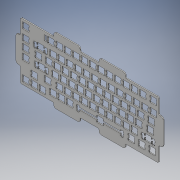
# Autodesk Inventor part: plate
Saved by Autodesk Inventor 2017 (Build 210142000, 142)
## iProperties
Created: 2021-06-16
Part Number: plate
Material: Generic
Document SubType Name: Modeling
Designer: Jack
Density: 1 g/cm^3
Appearance: Default
Author: Jack
Autodesk Inventor part; units mm, degrees
(part 1 of 3)
ref_plane "YZ Plane" through (0, 0, 0) normal (1, 0, 0) x (0, 1, 0)
ref_plane "XZ Plane" through (0, 0, 0) normal (0, 1, 0) x (-1, 0, 0)
ref_plane "XY Plane" through (0, 0, 0) normal (0, 0, 1) x (1, 0, 0)
sketch "Sketch1" plane through (0, 0, 0) normal (0, 1, 0) x (-1, 0, 0)
  line L0 (-149.0682, 63.7581) -> (-78.3822, 63.7581)
  line L1 (163.5067, 60.7579) -> (163.5067, 31.3429)
  line L2 (-152.0562, -63.0674) -> (-152.0562, -33.6571)
  line L3 (143.9807, -46.542) -> (143.9807, -47.5424)
  line L4 (143.9807, -47.5424) -> (143.1797, -47.5424)
  line L5 (143.1797, -47.5424) -> (143.1797, -50.6403)
  line L6 (143.1797, -50.6403) -> (143.9807, -50.6403)
  line L7 (143.9807, -50.6403) -> (143.9807, -56.4418)
  line L8 (143.9807, -56.4418) -> (143.1797, -56.4418)
  line L9 (143.1797, -56.4418) -> (143.1797, -59.5424)
  line L10 (143.1797, -59.5424) -> (143.9807, -59.5424)
  line L11 (143.9807, -59.5424) -> (143.9807, -60.5415)
  line L12 (143.9807, -60.5415) -> (157.9807, -60.5415)
  line L13 (157.9807, -60.5415) -> (157.9807, -59.5424)
  line L14 (157.9807, -59.5424) -> (158.7797, -59.5424)
  line L15 (158.7797, -59.5424) -> (158.7797, -56.4418)
  line L16 (158.7797, -56.4418) -> (157.9807, -56.4418)
  line L17 (157.9807, -56.4418) -> (157.9807, -50.6403)
  line L18 (157.9807, -50.6403) -> (158.7797, -50.6403)
  line L19 (158.7797, -50.6403) -> (158.7797, -47.5424)
  line L20 (158.7797, -47.5424) -> (157.9807, -47.5424)
  line L21 (157.9807, -47.5424) -> (157.9807, -46.542)
  line L22 (157.9807, -46.542) -> (143.9807, -46.542)
  line L23 (124.9307, -46.542) -> (124.9307, -47.5424)
  line L24 (124.9307, -47.5424) -> (124.1297, -47.5424)
  line L25 (124.1297, -47.5424) -> (124.1297, -50.6403)
  line L26 (124.1297, -50.6403) -> (124.9307, -50.6403)
  line L27 (124.9307, -50.6403) -> (124.9307, -56.4418)
  line L28 (124.9307, -56.4418) -> (124.1297, -56.4418)
  line L29 (124.1297, -56.4418) -> (124.1297, -59.5424)
  line L30 (124.1297, -59.5424) -> (124.9307, -59.5424)
  line L31 (124.9307, -59.5424) -> (124.9307, -60.5415)
  line L32 (124.9307, -60.5415) -> (138.9307, -60.5415)
  line L33 (138.9307, -60.5415) -> (138.9307, -59.5424)
  line L34 (138.9307, -59.5424) -> (139.7297, -59.5424)
  line L35 (139.7297, -59.5424) -> (139.7297, -56.4418)
  line L36 (139.7297, -56.4418) -> (138.9307, -56.4418)
  line L37 (138.9307, -56.4418) -> (138.9307, -50.6403)
  line L38 (138.9307, -50.6403) -> (139.7297, -50.6403)
  line L39 (139.7297, -50.6403) -> (139.7297, -47.5424)
  line L40 (139.7297, -47.5424) -> (138.9307, -47.5424)
  line L41 (138.9307, -47.5424) -> (138.9307, -46.542)
  line L42 (138.9307, -46.542) -> (124.9307, -46.542)
  line L43 (105.8807, -46.542) -> (105.8807, -47.5424)
  line L44 (105.8807, -47.5424) -> (105.0797, -47.5424)
  line L45 (105.0797, -47.5424) -> (105.0797, -50.6403)
  line L46 (105.0797, -50.6403) -> (105.8807, -50.6403)
  line L47 (105.8807, -50.6403) -> (105.8807, -56.4418)
  line L48 (105.8807, -56.4418) -> (105.0797, -56.4418)
  line L49 (105.0797, -56.4418) -> (105.0797, -59.5424)
  line L50 (105.0797, -59.5424) -> (105.8807, -59.5424)
  line L51 (105.8807, -59.5424) -> (105.8807, -60.5415)
  line L52 (105.8807, -60.5415) -> (119.8807, -60.5415)
  line L53 (119.8807, -60.5415) -> (119.8807, -59.5424)
  line L54 (119.8807, -59.5424) -> (120.6797, -59.5424)
  line L55 (120.6797, -59.5424) -> (120.6797, -56.4418)
  line L56 (120.6797, -56.4418) -> (119.8807, -56.4418)
  line L57 (119.8807, -56.4418) -> (119.8807, -50.6403)
  line L58 (119.8807, -50.6403) -> (120.6797, -50.6403)
  line L59 (120.6797, -50.6403) -> (120.6797, -47.5424)
  line L60 (120.6797, -47.5424) -> (119.8807, -47.5424)
  line L61 (119.8807, -47.5424) -> (119.8807, -46.542)
  line L62 (119.8807, -46.542) -> (105.8807, -46.542)
  line L63 (-25.0893, -41.7795) -> (-25.0893, -42.7785)
  line L64 (-25.0893, -42.7785) -> (-25.8883, -42.7785)
  line L65 (-25.8883, -42.7785) -> (-25.8883, -45.8791)
  line L66 (-25.8883, -45.8791) -> (-25.0893, -45.8791)
  line L67 (-25.0893, -45.8791) -> (-25.0893, -46.4786)
  line L68 (-25.0893, -46.4786) -> (-64.7132, -46.4786)
  line L69 (-64.7132, -46.4786) -> (-64.7132, -43.2484)
  line L70 (-64.7132, -43.2484) -> (-71.4643, -43.2484)
  line L71 (-71.4643, -43.2484) -> (-71.4643, -46.4786)
  line L72 (-71.4643, -46.4786) -> (-72.2884, -46.4786)
  line L73 (-72.2884, -46.4786) -> (-72.2884, -49.2788)
  line L74 (-72.2884, -49.2788) -> (-71.4643, -49.2788)
  line L75 (-71.4643, -49.2788) -> (-71.4643, -55.5488)
  line L76 (-71.4643, -55.5488) -> (-69.7393, -55.5488)
  line L77 (-69.7393, -55.5488) -> (-69.7393, -56.7491)
  line L78 (-69.7393, -56.7491) -> (-66.4387, -56.7491)
  line L79 (-66.4387, -56.7491) -> (-66.4387, -55.5488)
  line L80 (-66.4387, -55.5488) -> (-64.7132, -55.5488)
  line L81 (-64.7132, -55.5488) -> (-64.7132, -51.0785)
  line L82 (-64.7132, -51.0785) -> (-25.0893, -51.0785)
  line L83 (-25.0893, -51.0785) -> (-25.0893, -51.6793)
  line L84 (-25.0893, -51.6793) -> (-25.8883, -51.6793)
  line L85 (-25.8883, -51.6793) -> (-25.8883, -54.7785)
  line L86 (-25.8883, -54.7785) -> (-25.0893, -54.7785)
  line L87 (-25.0893, -54.7785) -> (-25.0893, -55.779)
  line L88 (-25.0893, -55.779) -> (-11.0883, -55.779)
  line L89 (-11.0883, -55.779) -> (-11.0883, -54.7785)
  line L90 (-11.0883, -54.7785) -> (-10.2893, -54.7785)
  line L91 (-10.2893, -54.7785) -> (-10.2893, -51.6793)
  line L92 (-10.2893, -51.6793) -> (-11.0883, -51.6793)
  line L93 (-11.0883, -51.6793) -> (-11.0883, -51.0785)
  line L94 (-11.0883, -51.0785) -> (28.5357, -51.0785)
  line L95 (28.5357, -51.0785) -> (28.5357, -55.5488)
  line L96 (28.5357, -55.5488) -> (30.2607, -55.5488)
  line L97 (30.2607, -55.5488) -> (30.2607, -56.7491)
  line L98 (30.2607, -56.7491) -> (33.5617, -56.7491)
  line L99 (33.5617, -56.7491) -> (33.5617, -55.5488)
  line L100 (33.5617, -55.5488) -> (35.2867, -55.5488)
  line L101 (35.2867, -55.5488) -> (35.2867, -49.2788)
  line L102 (35.2867, -49.2788) -> (36.1107, -49.2788)
  line L103 (36.1107, -49.2788) -> (36.1107, -46.4786)
  line L104 (36.1107, -46.4786) -> (35.2867, -46.4786)
  line L105 (35.2867, -46.4786) -> (35.2867, -43.2484)
  line L106 (35.2867, -43.2484) -> (28.5357, -43.2484)
  line L107 (28.5357, -43.2484) -> (28.5357, -46.4786)
  line L108 (28.5357, -46.4786) -> (-11.0883, -46.4786)
  line L109 (-11.0883, -46.4786) -> (-11.0883, -45.8791)
  line L110 (-11.0883, -45.8791) -> (-10.2893, -45.8791)
  line L111 (-10.2893, -45.8791) -> (-10.2893, -42.7785)
  line L112 (-10.2893, -42.7785) -> (-11.0883, -42.7785)
  line L113 (-11.0883, -42.7785) -> (-11.0883, -41.7795)
  line L114 (-11.0883, -41.7795) -> (-25.0893, -41.7795)
  line L115 (82.0687, -41.7795) -> (82.0687, -42.7785)
  line L116 (82.0687, -42.7785) -> (81.2677, -42.7785)
  line L117 (81.2677, -42.7785) -> (81.2677, -45.8791)
  line L118 (81.2677, -45.8791) -> (82.0687, -45.8791)
  line L119 (82.0687, -45.8791) -> (82.0687, -51.6793)
  line L120 (82.0687, -51.6793) -> (81.2677, -51.6793)
  line L121 (81.2677, -51.6793) -> (81.2677, -54.7785)
  line L122 (81.2677, -54.7785) -> (82.0687, -54.7785)
  line L123 (82.0687, -54.7785) -> (82.0687, -55.779)
  line L124 (82.0687, -55.779) -> (96.0677, -55.779)
  line L125 (96.0677, -55.779) -> (96.0677, -54.7785)
  line L126 (96.0677, -54.7785) -> (96.8687, -54.7785)
  line L127 (96.8687, -54.7785) -> (96.8687, -51.6793)
  line L128 (96.8687, -51.6793) -> (96.0677, -51.6793)
  line L129 (96.0677, -51.6793) -> (96.0677, -45.8791)
  line L130 (96.0677, -45.8791) -> (96.8687, -45.8791)
  line L131 (96.8687, -45.8791) -> (96.8687, -42.7785)
  line L132 (96.8687, -42.7785) -> (96.0677, -42.7785)
  line L133 (96.0677, -42.7785) -> (96.0677, -41.7795)
  line L134 (96.0677, -41.7795) -> (82.0687, -41.7795)
  line L135 (63.0187, -41.7795) -> (63.0187, -42.7785)
  line L136 (63.0187, -42.7785) -> (62.2177, -42.7785)
  line L137 (62.2177, -42.7785) -> (62.2177, -45.8791)
  line L138 (62.2177, -45.8791) -> (63.0187, -45.8791)
  line L139 (63.0187, -45.8791) -> (63.0187, -51.6793)
  line L140 (63.0187, -51.6793) -> (62.2177, -51.6793)
  line L141 (62.2177, -51.6793) -> (62.2177, -54.7785)
  line L142 (62.2177, -54.7785) -> (63.0187, -54.7785)
  line L143 (63.0187, -54.7785) -> (63.0187, -55.779)
  line L144 (63.0187, -55.779) -> (77.0177, -55.779)
  line L145 (77.0177, -55.779) -> (77.0177, -54.7785)
  line L146 (77.0177, -54.7785) -> (77.8187, -54.7785)
  line L147 (77.8187, -54.7785) -> (77.8187, -51.6793)
  line L148 (77.8187, -51.6793) -> (77.0177, -51.6793)
  line L149 (77.0177, -51.6793) -> (77.0177, -45.8791)
  line L150 (77.0177, -45.8791) -> (77.8187, -45.8791)
  line L151 (77.8187, -45.8791) -> (77.8187, -42.7785)
  line L152 (77.8187, -42.7785) -> (77.0177, -42.7785)
  line L153 (77.0177, -42.7785) -> (77.0177, -41.7795)
  line L154 (77.0177, -41.7795) -> (63.0187, -41.7795)
  line L155 (43.9687, -41.7795) -> (43.9687, -42.7785)
  line L156 (43.9687, -42.7785) -> (43.1677, -42.7785)
  line L157 (43.1677, -42.7785) -> (43.1677, -45.8791)
  line L158 (43.1677, -45.8791) -> (43.9687, -45.8791)
  line L159 (43.9687, -45.8791) -> (43.9687, -51.6793)
  line L160 (43.9687, -51.6793) -> (43.1677, -51.6793)
  line L161 (43.1677, -51.6793) -> (43.1677, -54.7785)
  line L162 (43.1677, -54.7785) -> (43.9687, -54.7785)
  line L163 (43.9687, -54.7785) -> (43.9687, -55.779)
  line L164 (43.9687, -55.779) -> (57.9677, -55.779)
  line L165 (57.9677, -55.779) -> (57.9677, -54.7785)
  line L166 (57.9677, -54.7785) -> (58.7687, -54.7785)
  line L167 (58.7687, -54.7785) -> (58.7687, -51.6793)
  line L168 (58.7687, -51.6793) -> (57.9677, -51.6793)
  line L169 (57.9677, -51.6793) -> (57.9677, -45.8791)
  line L170 (57.9677, -45.8791) -> (58.7687, -45.8791)
  line L171 (58.7687, -45.8791) -> (58.7687, -42.7785)
  line L172 (58.7687, -42.7785) -> (57.9677, -42.7785)
  line L173 (57.9677, -42.7785) -> (57.9677, -41.7795)
  line L174 (57.9677, -41.7795) -> (43.9687, -41.7795)
  line L175 (-96.5253, -41.7795) -> (-96.5253, -42.7785)
  line L176 (-96.5253, -42.7785) -> (-97.3261, -42.7785)
  line L177 (-97.3261, -42.7785) -> (-97.3261, -45.8791)
  line L178 (-97.3261, -45.8791) -> (-96.5253, -45.8791)
  line L179 (-96.5253, -45.8791) -> (-96.5253, -51.6793)
  line L180 (-96.5253, -51.6793) -> (-97.3261, -51.6793)
  line L181 (-97.3261, -51.6793) -> (-97.3261, -54.7785)
  line L182 (-97.3261, -54.7785) -> (-96.5253, -54.7785)
  line L183 (-96.5253, -54.7785) -> (-96.5253, -55.779)
  line L184 (-96.5253, -55.779) -> (-82.526, -55.779)
  line L185 (-82.526, -55.779) -> (-82.526, -54.7785)
  line L186 (-82.526, -54.7785) -> (-81.7252, -54.7785)
  line L187 (-81.7252, -54.7785) -> (-81.7252, -51.6793)
  line L188 (-81.7252, -51.6793) -> (-82.526, -51.6793)
  line L189 (-82.526, -51.6793) -> (-82.526, -45.8791)
  line L190 (-82.526, -45.8791) -> (-81.7252, -45.8791)
  line L191 (-81.7252, -45.8791) -> (-81.7252, -42.7785)
  line L192 (-81.7252, -42.7785) -> (-82.526, -42.7785)
  line L193 (-82.526, -42.7785) -> (-82.526, -41.7795)
  line L194 (-82.526, -41.7795) -> (-96.5253, -41.7795)
  line L195 (-120.3393, -41.7795) -> (-120.3393, -42.7785)
  line L196 (-120.3393, -42.7785) -> (-121.1385, -42.7785)
  line L197 (-121.1385, -42.7785) -> (-121.1385, -45.8791)
  line L198 (-121.1385, -45.8791) -> (-120.3393, -45.8791)
  line L199 (-120.3393, -45.8791) -> (-120.3393, -51.6793)
  line L200 (-120.3393, -51.6793) -> (-121.1385, -51.6793)
  line L201 (-121.1385, -51.6793) -> (-121.1385, -54.7785)
  line L202 (-121.1385, -54.7785) -> (-120.3393, -54.7785)
  line L203 (-120.3393, -54.7785) -> (-120.3393, -55.779)
  line L204 (-120.3393, -55.779) -> (-106.3385, -55.779)
  line L205 (-106.3385, -55.779) -> (-106.3385, -54.7785)
  line L206 (-106.3385, -54.7785) -> (-105.5391, -54.7785)
  line L207 (-105.5391, -54.7785) -> (-105.5391, -51.6793)
  line L208 (-105.5391, -51.6793) -> (-106.3385, -51.6793)
  line L209 (-106.3385, -51.6793) -> (-106.3385, -45.8791)
  line L210 (-106.3385, -45.8791) -> (-105.5391, -45.8791)
  line L211 (-105.5391, -45.8791) -> (-105.5391, -42.7785)
  line L212 (-105.5391, -42.7785) -> (-106.3385, -42.7785)
  line L213 (-106.3385, -42.7785) -> (-106.3385, -41.7795)
  line L214 (-106.3385, -41.7795) -> (-120.3393, -41.7795)
  line L215 (-144.1504, -41.7795) -> (-144.1504, -42.7785)
  line L216 (-144.1504, -42.7785) -> (-144.951, -42.7785)
  line L217 (-144.951, -42.7785) -> (-144.951, -45.8791)
  line L218 (-144.951, -45.8791) -> (-144.1504, -45.8791)
  line L219 (-144.1504, -45.8791) -> (-144.1504, -51.6793)
  line L220 (-144.1504, -51.6793) -> (-144.951, -51.6793)
  line L221 (-144.951, -51.6793) -> (-144.951, -54.7785)
  line L222 (-144.951, -54.7785) -> (-144.1504, -54.7785)
  line L223 (-144.1504, -54.7785) -> (-144.1504, -55.779)
  line L224 (-144.1504, -55.779) -> (-130.1509, -55.779)
  line L225 (-130.1509, -55.779) -> (-130.1509, -54.7785)
  line L226 (-130.1509, -54.7785) -> (-129.3503, -54.7785)
  line L227 (-129.3503, -54.7785) -> (-129.3503, -51.6793)
  line L228 (-129.3503, -51.6793) -> (-130.1509, -51.6793)
  line L229 (-130.1509, -51.6793) -> (-130.1509, -45.8791)
  line L230 (-130.1509, -45.8791) -> (-129.3503, -45.8791)
  line L231 (-129.3503, -45.8791) -> (-129.3503, -42.7785)
  line L232 (-129.3503, -42.7785) -> (-130.1509, -42.7785)
  line L233 (-130.1509, -42.7785) -> (-130.1509, -41.7795)
  line L234 (-130.1509, -41.7795) -> (-144.1504, -41.7795)
  line L235 (124.9307, -27.4921) -> (124.9307, -28.4924)
  line L236 (124.9307, -28.4924) -> (124.1297, -28.4924)
  line L237 (124.1297, -28.4924) -> (124.1297, -31.5916)
  line L238 (124.1297, -31.5916) -> (124.9307, -31.5916)
  line L239 (124.9307, -31.5916) -> (124.9307, -37.3918)
  line L240 (124.9307, -37.3918) -> (124.1297, -37.3918)
  line L241 (124.1297, -37.3918) -> (124.1297, -40.4924)
  line L242 (124.1297, -40.4924) -> (124.9307, -40.4924)
  line L243 (124.9307, -40.4924) -> (124.9307, -41.4915)
  line L244 (124.9307, -41.4915) -> (138.9307, -41.4915)
  line L245 (138.9307, -41.4915) -> (138.9307, -40.4924)
  line L246 (138.9307, -40.4924) -> (139.7297, -40.4924)
  line L247 (139.7297, -40.4924) -> (139.7297, -37.3918)
  line L248 (139.7297, -37.3918) -> (138.9307, -37.3918)
  line L249 (138.9307, -37.3918) -> (138.9307, -31.5916)
  line L250 (138.9307, -31.5916) -> (139.7297, -31.5916)
  line L251 (139.7297, -31.5916) -> (139.7297, -28.4924)
  line L252 (139.7297, -28.4924) -> (138.9307, -28.4924)
  line L253 (138.9307, -28.4924) -> (138.9307, -27.4921)
  line L254 (138.9307, -27.4921) -> (124.9307, -27.4921)
  line L255 (-134.6254, -22.7296) -> (-134.6254, -23.7286)
  line L256 (-134.6254, -23.7286) -> (-135.426, -23.7286)
  line L257 (-135.426, -23.7286) -> (-135.426, -26.8292)
  line L258 (-135.426, -26.8292) -> (-134.6254, -26.8292)
  line L259 (-134.6254, -26.8292) -> (-134.6254, -27.4286)
  line L260 (-134.6254, -27.4286) -> (-136.1509, -27.4286)
  line L261 (-136.1509, -27.4286) -> (-136.1509, -24.1985)
  line L262 (-136.1509, -24.1985) -> (-142.9005, -24.1985)
  line L263 (-142.9005, -24.1985) -> (-142.9005, -27.4286)
  line L264 (-142.9005, -27.4286) -> (-143.726, -27.4286)
  line L265 (-143.726, -27.4286) -> (-143.726, -30.2288)
  line L266 (-143.726, -30.2288) -> (-142.9005, -30.2288)
  line L267 (-142.9005, -30.2288) -> (-142.9005, -36.4988)
  line L268 (-142.9005, -36.4988) -> (-141.1752, -36.4988)
  line L269 (-141.1752, -36.4988) -> (-141.1752, -37.6991)
  line L270 (-141.1752, -37.6991) -> (-137.8762, -37.6991)
  line L271 (-137.8762, -37.6991) -> (-137.8762, -36.4988)
  line L272 (-137.8762, -36.4988) -> (-136.1509, -36.4988)
  line L273 (-136.1509, -36.4988) -> (-136.1509, -32.0285)
  line L274 (-136.1509, -32.0285) -> (-134.6254, -32.0285)
  line L275 (-134.6254, -32.0285) -> (-134.6254, -32.6293)
  line L276 (-134.6254, -32.6293) -> (-135.426, -32.6293)
  line L277 (-135.426, -32.6293) -> (-135.426, -35.7285)
  line L278 (-135.426, -35.7285) -> (-134.6254, -35.7285)
  line L279 (-134.6254, -35.7285) -> (-134.6254, -36.729)
  line L280 (-134.6254, -36.729) -> (-120.6259, -36.729)
  line L281 (-120.6259, -36.729) -> (-120.6259, -35.7285)
  line L282 (-120.6259, -35.7285) -> (-119.8253, -35.7285)
  line L283 (-119.8253, -35.7285) -> (-119.8253, -32.6293)
  line L284 (-119.8253, -32.6293) -> (-120.6259, -32.6293)
  line L285 (-120.6259, -32.6293) -> (-120.6259, -32.0285)
  line L286 (-120.6259, -32.0285) -> (-119.1004, -32.0285)
  line L287 (-119.1004, -32.0285) -> (-119.1004, -36.4988)
  line L288 (-119.1004, -36.4988) -> (-117.3765, -36.4988)
  line L289 (-117.3765, -36.4988) -> (-117.3765, -37.6991)
  line L290 (-117.3765, -37.6991) -> (-114.0761, -37.6991)
  line L291 (-114.0761, -37.6991) -> (-114.0761, -36.4988)
  line L292 (-114.0761, -36.4988) -> (-112.3509, -36.4988)
  line L293 (-112.3509, -36.4988) -> (-112.3509, -30.2288)
  line L294 (-112.3509, -30.2288) -> (-111.5254, -30.2288)
  line L295 (-111.5254, -30.2288) -> (-111.5254, -27.4286)
  line L296 (-111.5254, -27.4286) -> (-112.3509, -27.4286)
  line L297 (-112.3509, -27.4286) -> (-112.3509, -24.1985)
  line L298 (-112.3509, -24.1985) -> (-119.1004, -24.1985)
  line L299 (-119.1004, -24.1985) -> (-119.1004, -27.4286)
  line L300 (-119.1004, -27.4286) -> (-120.6259, -27.4286)
  line L301 (-120.6259, -27.4286) -> (-120.6259, -26.8292)
  line L302 (-120.6259, -26.8292) -> (-119.8253, -26.8292)
  line L303 (-119.8253, -26.8292) -> (-119.8253, -23.7286)
  line L304 (-119.8253, -23.7286) -> (-120.6259, -23.7286)
  line L305 (-120.6259, -23.7286) -> (-120.6259, -22.7296)
  line L306 (-120.6259, -22.7296) -> (-134.6254, -22.7296)
  line L307 (93.9747, -22.7296) -> (93.9747, -23.7286)
  line L308 (93.9747, -23.7286) -> (93.1737, -23.7286)
  line L309 (93.1737, -23.7286) -> (93.1737, -26.8292)
  line L310 (93.1737, -26.8292) -> (93.9747, -26.8292)
  line L311 (93.9747, -26.8292) -> (93.9747, -32.6293)
  line L312 (93.9747, -32.6293) -> (93.1737, -32.6293)
  line L313 (93.1737, -32.6293) -> (93.1737, -35.7285)
  line L314 (93.1737, -35.7285) -> (93.9747, -35.7285)
  line L315 (93.9747, -35.7285) -> (93.9747, -36.729)
  line L316 (93.9747, -36.729) -> (107.9737, -36.729)
  line L317 (107.9737, -36.729) -> (107.9737, -35.7285)
  line L318 (107.9737, -35.7285) -> (108.7747, -35.7285)
  line L319 (108.7747, -35.7285) -> (108.7747, -32.6293)
  line L320 (108.7747, -32.6293) -> (107.9737, -32.6293)
  line L321 (107.9737, -32.6293) -> (107.9737, -26.8292)
  line L322 (107.9737, -26.8292) -> (108.7747, -26.8292)
  line L323 (108.7747, -26.8292) -> (108.7747, -23.7286)
  line L324 (108.7747, -23.7286) -> (107.9737, -23.7286)
  line L325 (107.9737, -23.7286) -> (107.9737, -22.7296)
  line L326 (107.9737, -22.7296) -> (93.9747, -22.7296)
  line L327 (67.7807, -22.7296) -> (67.7807, -23.7286)
  line L328 (67.7807, -23.7286) -> (66.9797, -23.7286)
  line L329 (66.9797, -23.7286) -> (66.9797, -26.8292)
  line L330 (66.9797, -26.8292) -> (67.7807, -26.8292)
  line L331 (67.7807, -26.8292) -> (67.7807, -32.6293)
  line L332 (67.7807, -32.6293) -> (66.9797, -32.6293)
  line L333 (66.9797, -32.6293) -> (66.9797, -35.7285)
  line L334 (66.9797, -35.7285) -> (67.7807, -35.7285)
  line L335 (67.7807, -35.7285) -> (67.7807, -36.729)
  line L336 (67.7807, -36.729) -> (81.7807, -36.729)
  line L337 (81.7807, -36.729) -> (81.7807, -35.7285)
  line L338 (81.7807, -35.7285) -> (82.5797, -35.7285)
  line L339 (82.5797, -35.7285) -> (82.5797, -32.6293)
  line L340 (82.5797, -32.6293) -> (81.7807, -32.6293)
  line L341 (81.7807, -32.6293) -> (81.7807, -26.8292)
  line L342 (81.7807, -26.8292) -> (82.5797, -26.8292)
  line L343 (82.5797, -26.8292) -> (82.5797, -23.7286)
  line L344 (82.5797, -23.7286) -> (81.7807, -23.7286)
  line L345 (81.7807, -23.7286) -> (81.7807, -22.7296)
  line L346 (81.7807, -22.7296) -> (67.7807, -22.7296)
  line L347 (48.7307, -22.7296) -> (48.7307, -23.7286)
  line L348 (48.7307, -23.7286) -> (47.9297, -23.7286)
  line L349 (47.9297, -23.7286) -> (47.9297, -26.8292)
  line L350 (47.9297, -26.8292) -> (48.7307, -26.8292)
  line L351 (48.7307, -26.8292) -> (48.7307, -32.6293)
  line L352 (48.7307, -32.6293) -> (47.9297, -32.6293)
  line L353 (47.9297, -32.6293) -> (47.9297, -35.7285)
  line L354 (47.9297, -35.7285) -> (48.7307, -35.7285)
  line L355 (48.7307, -35.7285) -> (48.7307, -36.729)
  line L356 (48.7307, -36.729) -> (62.7307, -36.729)
  line L357 (62.7307, -36.729) -> (62.7307, -35.7285)
  line L358 (62.7307, -35.7285) -> (63.5297, -35.7285)
  line L359 (63.5297, -35.7285) -> (63.5297, -32.6293)
  line L360 (63.5297, -32.6293) -> (62.7307, -32.6293)
  line L361 (62.7307, -32.6293) -> (62.7307, -26.8292)
  line L362 (62.7307, -26.8292) -> (63.5297, -26.8292)
  line L363 (63.5297, -26.8292) -> (63.5297, -23.7286)
  line L364 (63.5297, -23.7286) -> (62.7307, -23.7286)
  line L365 (62.7307, -23.7286) -> (62.7307, -22.7296)
  line L366 (62.7307, -22.7296) -> (48.7307, -22.7296)
  line L367 (29.6807, -22.7296) -> (29.6807, -23.7286)
  line L368 (29.6807, -23.7286) -> (28.8797, -23.7286)
  line L369 (28.8797, -23.7286) -> (28.8797, -26.8292)
  line L370 (28.8797, -26.8292) -> (29.6807, -26.8292)
  line L371 (29.6807, -26.8292) -> (29.6807, -32.6293)
  line L372 (29.6807, -32.6293) -> (28.8797, -32.6293)
  line L373 (28.8797, -32.6293) -> (28.8797, -35.7285)
  line L374 (28.8797, -35.7285) -> (29.6807, -35.7285)
  line L375 (29.6807, -35.7285) -> (29.6807, -36.729)
  line L376 (29.6807, -36.729) -> (43.6807, -36.729)
  line L377 (43.6807, -36.729) -> (43.6807, -35.7285)
  line L378 (43.6807, -35.7285) -> (44.4797, -35.7285)
  line L379 (44.4797, -35.7285) -> (44.4797, -32.6293)
  line L380 (44.4797, -32.6293) -> (43.6807, -32.6293)
  line L381 (43.6807, -32.6293) -> (43.6807, -26.8292)
  line L382 (43.6807, -26.8292) -> (44.4797, -26.8292)
  line L383 (44.4797, -26.8292) -> (44.4797, -23.7286)
  line L384 (44.4797, -23.7286) -> (43.6807, -23.7286)
  line L385 (43.6807, -23.7286) -> (43.6807, -22.7296)
  line L386 (43.6807, -22.7296) -> (29.6807, -22.7296)
  line L387 (10.6307, -22.7296) -> (10.6307, -23.7286)
  line L388 (10.6307, -23.7286) -> (9.8297, -23.7286)
  line L389 (9.8297, -23.7286) -> (9.8297, -26.8292)
  line L390 (9.8297, -26.8292) -> (10.6307, -26.8292)
  line L391 (10.6307, -26.8292) -> (10.6307, -32.6293)
  line L392 (10.6307, -32.6293) -> (9.8297, -32.6293)
  line L393 (9.8297, -32.6293) -> (9.8297, -35.7285)
  line L394 (9.8297, -35.7285) -> (10.6307, -35.7285)
  line L395 (10.6307, -35.7285) -> (10.6307, -36.729)
  line L396 (10.6307, -36.729) -> (24.6307, -36.729)
  line L397 (24.6307, -36.729) -> (24.6307, -35.7285)
  line L398 (24.6307, -35.7285) -> (25.4297, -35.7285)
  line L399 (25.4297, -35.7285) -> (25.4297, -32.6293)
  line L400 (25.4297, -32.6293) -> (24.6307, -32.6293)
  line L401 (24.6307, -32.6293) -> (24.6307, -26.8292)
  line L402 (24.6307, -26.8292) -> (25.4297, -26.8292)
  line L403 (25.4297, -26.8292) -> (25.4297, -23.7286)
  line L404 (25.4297, -23.7286) -> (24.6307, -23.7286)
  line L405 (24.6307, -23.7286) -> (24.6307, -22.7296)
  line L406 (24.6307, -22.7296) -> (10.6307, -22.7296)
  line L407 (-8.4193, -22.7296) -> (-8.4193, -23.7286)
  line L408 (-8.4193, -23.7286) -> (-9.2203, -23.7286)
  line L409 (-9.2203, -23.7286) -> (-9.2203, -26.8292)
  line L410 (-9.2203, -26.8292) -> (-8.4193, -26.8292)
  line L411 (-8.4193, -26.8292) -> (-8.4193, -32.6293)
  line L412 (-8.4193, -32.6293) -> (-9.2203, -32.6293)
  line L413 (-9.2203, -32.6293) -> (-9.2203, -35.7285)
  line L414 (-9.2203, -35.7285) -> (-8.4193, -35.7285)
  line L415 (-8.4193, -35.7285) -> (-8.4193, -36.729)
  line L416 (-8.4193, -36.729) -> (5.5807, -36.729)
  line L417 (5.5807, -36.729) -> (5.5807, -35.7285)
  line L418 (5.5807, -35.7285) -> (6.3797, -35.7285)
  line L419 (6.3797, -35.7285) -> (6.3797, -32.6293)
  line L420 (6.3797, -32.6293) -> (5.5807, -32.6293)
  line L421 (5.5807, -32.6293) -> (5.5807, -26.8292)
  line L422 (5.5807, -26.8292) -> (6.3797, -26.8292)
  line L423 (6.3797, -26.8292) -> (6.3797, -23.7286)
  line L424 (6.3797, -23.7286) -> (5.5807, -23.7286)
  line L425 (5.5807, -23.7286) -> (5.5807, -22.7296)
  line L426 (5.5807, -22.7296) -> (-8.4193, -22.7296)
  line L427 (-27.4693, -22.7296) -> (-27.4693, -23.7286)
  line L428 (-27.4693, -23.7286) -> (-28.2703, -23.7286)
  line L429 (-28.2703, -23.7286) -> (-28.2703, -26.8292)
  line L430 (-28.2703, -26.8292) -> (-27.4693, -26.8292)
  line L431 (-27.4693, -26.8292) -> (-27.4693, -32.6293)
  line L432 (-27.4693, -32.6293) -> (-28.2703, -32.6293)
  line L433 (-28.2703, -32.6293) -> (-28.2703, -35.7285)
  line L434 (-28.2703, -35.7285) -> (-27.4693, -35.7285)
  line L435 (-27.4693, -35.7285) -> (-27.4693, -36.729)
  line L436 (-27.4693, -36.729) -> (-13.4693, -36.729)
  line L437 (-13.4693, -36.729) -> (-13.4693, -35.7285)
  line L438 (-13.4693, -35.7285) -> (-12.6703, -35.7285)
  line L439 (-12.6703, -35.7285) -> (-12.6703, -32.6293)
  line L440 (-12.6703, -32.6293) -> (-13.4693, -32.6293)
  line L441 (-13.4693, -32.6293) -> (-13.4693, -26.8292)
  line L442 (-13.4693, -26.8292) -> (-12.6703, -26.8292)
  line L443 (-12.6703, -26.8292) -> (-12.6703, -23.7286)
  line L444 (-12.6703, -23.7286) -> (-13.4693, -23.7286)
  line L445 (-13.4693, -23.7286) -> (-13.4693, -22.7296)
  line L446 (-13.4693, -22.7296) -> (-27.4693, -22.7296)
  line L447 (-46.5193, -22.7296) -> (-46.5193, -23.7286)
  line L448 (-46.5193, -23.7286) -> (-47.3203, -23.7286)
  line L449 (-47.3203, -23.7286) -> (-47.3203, -26.8292)
  line L450 (-47.3203, -26.8292) -> (-46.5193, -26.8292)
  line L451 (-46.5193, -26.8292) -> (-46.5193, -32.6293)
  line L452 (-46.5193, -32.6293) -> (-47.3203, -32.6293)
  line L453 (-47.3203, -32.6293) -> (-47.3203, -35.7285)
  line L454 (-47.3203, -35.7285) -> (-46.5193, -35.7285)
  line L455 (-46.5193, -35.7285) -> (-46.5193, -36.729)
  line L456 (-46.5193, -36.729) -> (-32.5193, -36.729)
  line L457 (-32.5193, -36.729) -> (-32.5193, -35.7285)
  line L458 (-32.5193, -35.7285) -> (-31.7203, -35.7285)
  line L459 (-31.7203, -35.7285) -> (-31.7203, -32.6293)
  line L460 (-31.7203, -32.6293) -> (-32.5193, -32.6293)
  line L461 (-32.5193, -32.6293) -> (-32.5193, -26.8292)
  line L462 (-32.5193, -26.8292) -> (-31.7203, -26.8292)
  line L463 (-31.7203, -26.8292) -> (-31.7203, -23.7286)
  line L464 (-31.7203, -23.7286) -> (-32.5193, -23.7286)
  line L465 (-32.5193, -23.7286) -> (-32.5193, -22.7296)
  line L466 (-32.5193, -22.7296) -> (-46.5193, -22.7296)
  line L467 (-65.5691, -22.7296) -> (-65.5691, -23.7286)
  line L468 (-65.5691, -23.7286) -> (-66.3699, -23.7286)
  line L469 (-66.3699, -23.7286) -> (-66.3699, -26.8292)
  line L470 (-66.3699, -26.8292) -> (-65.5691, -26.8292)
  line L471 (-65.5691, -26.8292) -> (-65.5691, -32.6293)
  line L472 (-65.5691, -32.6293) -> (-66.3699, -32.6293)
  line L473 (-66.3699, -32.6293) -> (-66.3699, -35.7285)
  line L474 (-66.3699, -35.7285) -> (-65.5691, -35.7285)
  line L475 (-65.5691, -35.7285) -> (-65.5691, -36.729)
  line L476 (-65.5691, -36.729) -> (-51.5698, -36.729)
  line L477 (-51.5698, -36.729) -> (-51.5698, -35.7285)
  line L478 (-51.5698, -35.7285) -> (-50.7704, -35.7285)
  line L479 (-50.7704, -35.7285) -> (-50.7704, -32.6293)
  line L480 (-50.7704, -32.6293) -> (-51.5698, -32.6293)
  line L481 (-51.5698, -32.6293) -> (-51.5698, -26.8292)
  line L482 (-51.5698, -26.8292) -> (-50.7704, -26.8292)
  line L483 (-50.7704, -26.8292) -> (-50.7704, -23.7286)
  line L484 (-50.7704, -23.7286) -> (-51.5698, -23.7286)
  line L485 (-51.5698, -23.7286) -> (-51.5698, -22.7296)
  line L486 (-51.5698, -22.7296) -> (-65.5691, -22.7296)
  line L487 (-84.6191, -22.7296) -> (-84.6191, -23.7286)
  line L488 (-84.6191, -23.7286) -> (-85.4199, -23.7286)
  line L489 (-85.4199, -23.7286) -> (-85.4199, -26.8292)
  line L490 (-85.4199, -26.8292) -> (-84.6191, -26.8292)
  line L491 (-84.6191, -26.8292) -> (-84.6191, -32.6293)
  line L492 (-84.6191, -32.6293) -> (-85.4199, -32.6293)
  line L493 (-85.4199, -32.6293) -> (-85.4199, -35.7285)
  line L494 (-85.4199, -35.7285) -> (-84.6191, -35.7285)
  line L495 (-84.6191, -35.7285) -> (-84.6191, -36.729)
  line L496 (-84.6191, -36.729) -> (-70.6198, -36.729)
  line L497 (-70.6198, -36.729) -> (-70.6198, -35.7285)
  line L498 (-70.6198, -35.7285) -> (-69.8204, -35.7285)
  line L499 (-69.8204, -35.7285) -> (-69.8204, -32.6293)
  line L500 (-69.8204, -32.6293) -> (-70.6198, -32.6293)
  line L501 (-70.6198, -32.6293) -> (-70.6198, -26.8292)
  line L502 (-70.6198, -26.8292) -> (-69.8204, -26.8292)
  line L503 (-69.8204, -26.8292) -> (-69.8204, -23.7286)
  line L504 (-69.8204, -23.7286) -> (-70.6198, -23.7286)
  line L505 (-70.6198, -23.7286) -> (-70.6198, -22.7296)
  line L506 (-70.6198, -22.7296) -> (-84.6191, -22.7296)
  line L507 (-103.6691, -22.7296) -> (-103.6691, -23.7286)
  line L508 (-103.6691, -23.7286) -> (-104.4699, -23.7286)
  line L509 (-104.4699, -23.7286) -> (-104.4699, -26.8292)
  line L510 (-104.4699, -26.8292) -> (-103.6691, -26.8292)
  line L511 (-103.6691, -26.8292) -> (-103.6691, -32.6293)
  line L512 (-103.6691, -32.6293) -> (-104.4699, -32.6293)
  line L513 (-104.4699, -32.6293) -> (-104.4699, -35.7285)
  line L514 (-104.4699, -35.7285) -> (-103.6691, -35.7285)
  line L515 (-103.6691, -35.7285) -> (-103.6691, -36.729)
  line L516 (-103.6691, -36.729) -> (-89.6698, -36.729)
  line L517 (-89.6698, -36.729) -> (-89.6698, -35.7285)
  line L518 (-89.6698, -35.7285) -> (-88.8704, -35.7285)
  line L519 (-88.8704, -35.7285) -> (-88.8704, -32.6293)
  line L520 (-88.8704, -32.6293) -> (-89.6698, -32.6293)
  line L521 (-89.6698, -32.6293) -> (-89.6698, -26.8292)
  line L522 (-89.6698, -26.8292) -> (-88.8704, -26.8292)
  line L523 (-88.8704, -26.8292) -> (-88.8704, -23.7286)
  line L524 (-88.8704, -23.7286) -> (-89.6698, -23.7286)
  line L525 (-89.6698, -23.7286) -> (-89.6698, -22.7296)
  line L526 (-89.6698, -22.7296) -> (-103.6691, -22.7296)
  line L527 (108.2607, -3.6795) -> (108.2607, -4.6786)
  line L528 (108.2607, -4.6786) -> (107.4597, -4.6786)
  line L529 (107.4597, -4.6786) -> (107.4597, -7.7792)
  line L530 (107.4597, -7.7792) -> (108.2607, -7.7792)
  line L531 (108.2607, -7.7792) -> (108.2607, -8.3786)
  line L532 (108.2607, -8.3786) -> (106.7367, -8.3786)
  line L533 (106.7367, -8.3786) -> (106.7367, -5.1485)
  line L534 (106.7367, -5.1485) -> (99.9857, -5.1485)
  line L535 (99.9857, -5.1485) -> (99.9857, -8.3786)
  line L536 (99.9857, -8.3786) -> (99.1617, -8.3786)
  line L537 (99.1617, -8.3786) -> (99.1617, -11.1789)
  line L538 (99.1617, -11.1789) -> (99.9857, -11.1789)
  line L539 (99.9857, -11.1789) -> (99.9857, -17.4488)
  line L540 (99.9857, -17.4488) -> (101.7107, -17.4488)
  line L541 (101.7107, -17.4488) -> (101.7107, -18.649)
  line L542 (101.7107, -18.649) -> (105.0097, -18.649)
  line L543 (105.0097, -18.649) -> (105.0097, -17.4488)
  line L544 (105.0097, -17.4488) -> (106.7367, -17.4488)
  line L545 (106.7367, -17.4488) -> (106.7367, -12.9784)
  line L546 (106.7367, -12.9784) -> (108.2607, -12.9784)
  line L547 (108.2607, -12.9784) -> (108.2607, -13.5792)
  line L548 (108.2607, -13.5792) -> (107.4597, -13.5792)
  line L549 (107.4597, -13.5792) -> (107.4597, -16.6784)
  line L550 (107.4597, -16.6784) -> (108.2607, -16.6784)
  line L551 (108.2607, -16.6784) -> (108.2607, -17.6788)
  line L552 (108.2607, -17.6788) -> (122.2617, -17.6788)
  line L553 (122.2617, -17.6788) -> (122.2617, -16.6784)
  line L554 (122.2617, -16.6784) -> (123.0607, -16.6784)
  line L555 (123.0607, -16.6784) -> (123.0607, -13.5792)
  line L556 (123.0607, -13.5792) -> (122.2617, -13.5792)
  line L557 (122.2617, -13.5792) -> (122.2617, -12.9784)
  line L558 (122.2617, -12.9784) -> (123.7857, -12.9784)
  line L559 (123.7857, -12.9784) -> (123.7857, -17.4488)
  line L560 (123.7857, -17.4488) -> (125.5107, -17.4488)
  line L561 (125.5107, -17.4488) -> (125.5107, -18.649)
  line L562 (125.5107, -18.649) -> (128.8117, -18.649)
  line L563 (128.8117, -18.649) -> (128.8117, -17.4488)
  line L564 (128.8117, -17.4488) -> (130.5367, -17.4488)
  line L565 (130.5367, -17.4488) -> (130.5367, -11.1789)
  line L566 (130.5367, -11.1789) -> (131.3607, -11.1789)
  line L567 (131.3607, -11.1789) -> (131.3607, -8.3786)
  line L568 (131.3607, -8.3786) -> (130.5367, -8.3786)
  line L569 (130.5367, -8.3786) -> (130.5367, -5.1485)
  line L570 (130.5367, -5.1485) -> (123.7857, -5.1485)
  line L571 (123.7857, -5.1485) -> (123.7857, -8.3786)
  line L572 (123.7857, -8.3786) -> (122.2617, -8.3786)
  line L573 (122.2617, -8.3786) -> (122.2617, -7.7792)
  line L574 (122.2617, -7.7792) -> (123.0607, -7.7792)
  line L575 (123.0607, -7.7792) -> (123.0607, -4.6786)
  line L576 (123.0607, -4.6786) -> (122.2617, -4.6786)
  line L577 (122.2617, -4.6786) -> (122.2617, -3.6795)
  line L578 (122.2617, -3.6795) -> (108.2607, -3.6795)
  line L579 (143.9807, -3.6795) -> (143.9807, -4.6786)
  line L580 (143.9807, -4.6786) -> (143.1797, -4.6786)
  line L581 (143.1797, -4.6786) -> (143.1797, -7.7792)
  line L582 (143.1797, -7.7792) -> (143.9807, -7.7792)
  line L583 (143.9807, -7.7792) -> (143.9807, -13.5792)
  line L584 (143.9807, -13.5792) -> (143.1797, -13.5792)
  line L585 (143.1797, -13.5792) -> (143.1797, -16.6784)
  line L586 (143.1797, -16.6784) -> (143.9807, -16.6784)
  line L587 (143.9807, -16.6784) -> (143.9807, -17.6788)
  line L588 (143.9807, -17.6788) -> (157.9807, -17.6788)
  line L589 (157.9807, -17.6788) -> (157.9807, -16.6784)
  line L590 (157.9807, -16.6784) -> (158.7797, -16.6784)
  line L591 (158.7797, -16.6784) -> (158.7797, -13.5792)
  line L592 (158.7797, -13.5792) -> (157.9807, -13.5792)
  line L593 (157.9807, -13.5792) -> (157.9807, -7.7792)
  line L594 (157.9807, -7.7792) -> (158.7797, -7.7792)
  line L595 (158.7797, -7.7792) -> (158.7797, -4.6786)
  line L596 (158.7797, -4.6786) -> (157.9807, -4.6786)
  line L597 (157.9807, -4.6786) -> (157.9807, -3.6795)
  line L598 (157.9807, -3.6795) -> (143.9807, -3.6795)
  line L599 (77.3057, -3.6795) -> (77.3057, -4.6786)
  line L600 (77.3057, -4.6786) -> (76.5047, -4.6786)
  line L601 (76.5047, -4.6786) -> (76.5047, -7.7792)
  line L602 (76.5047, -7.7792) -> (77.3057, -7.7792)
  line L603 (77.3057, -7.7792) -> (77.3057, -13.5792)
  line L604 (77.3057, -13.5792) -> (76.5047, -13.5792)
  line L605 (76.5047, -13.5792) -> (76.5047, -16.6784)
  line L606 (76.5047, -16.6784) -> (77.3057, -16.6784)
  line L607 (77.3057, -16.6784) -> (77.3057, -17.6788)
  line L608 (77.3057, -17.6788) -> (91.3057, -17.6788)
  line L609 (91.3057, -17.6788) -> (91.3057, -16.6784)
  line L610 (91.3057, -16.6784) -> (92.1047, -16.6784)
  line L611 (92.1047, -16.6784) -> (92.1047, -13.5792)
  line L612 (92.1047, -13.5792) -> (91.3057, -13.5792)
  line L613 (91.3057, -13.5792) -> (91.3057, -7.7792)
  line L614 (91.3057, -7.7792) -> (92.1047, -7.7792)
  line L615 (92.1047, -7.7792) -> (92.1047, -4.6786)
  line L616 (92.1047, -4.6786) -> (91.3057, -4.6786)
  line L617 (91.3057, -4.6786) -> (91.3057, -3.6795)
  line L618 (91.3057, -3.6795) -> (77.3057, -3.6795)
  line L619 (58.2557, -3.6795) -> (58.2557, -4.6786)
  line L620 (58.2557, -4.6786) -> (57.4547, -4.6786)
  line L621 (57.4547, -4.6786) -> (57.4547, -7.7792)
  line L622 (57.4547, -7.7792) -> (58.2557, -7.7792)
  line L623 (58.2557, -7.7792) -> (58.2557, -13.5792)
  line L624 (58.2557, -13.5792) -> (57.4547, -13.5792)
  line L625 (57.4547, -13.5792) -> (57.4547, -16.6784)
  line L626 (57.4547, -16.6784) -> (58.2557, -16.6784)
  line L627 (58.2557, -16.6784) -> (58.2557, -17.6788)
  line L628 (58.2557, -17.6788) -> (72.2557, -17.6788)
  line L629 (72.2557, -17.6788) -> (72.2557, -16.6784)
  line L630 (72.2557, -16.6784) -> (73.0547, -16.6784)
  line L631 (73.0547, -16.6784) -> (73.0547, -13.5792)
  line L632 (73.0547, -13.5792) -> (72.2557, -13.5792)
  line L633 (72.2557, -13.5792) -> (72.2557, -7.7792)
  line L634 (72.2557, -7.7792) -> (73.0547, -7.7792)
  line L635 (73.0547, -7.7792) -> (73.0547, -4.6786)
  line L636 (73.0547, -4.6786) -> (72.2557, -4.6786)
  line L637 (72.2557, -4.6786) -> (72.2557, -3.6795)
  line L638 (72.2557, -3.6795) -> (58.2557, -3.6795)
  line L639 (39.2057, -3.6795) -> (39.2057, -4.6786)
  line L640 (39.2057, -4.6786) -> (38.4047, -4.6786)
  line L641 (38.4047, -4.6786) -> (38.4047, -7.7792)
  line L642 (38.4047, -7.7792) -> (39.2057, -7.7792)
  line L643 (39.2057, -7.7792) -> (39.2057, -13.5792)
  line L644 (39.2057, -13.5792) -> (38.4047, -13.5792)
  line L645 (38.4047, -13.5792) -> (38.4047, -16.6784)
  line L646 (38.4047, -16.6784) -> (39.2057, -16.6784)
  line L647 (39.2057, -16.6784) -> (39.2057, -17.6788)
  line L648 (39.2057, -17.6788) -> (53.2057, -17.6788)
  line L649 (53.2057, -17.6788) -> (53.2057, -16.6784)
  line L650 (53.2057, -16.6784) -> (54.0047, -16.6784)
  line L651 (54.0047, -16.6784) -> (54.0047, -13.5792)
  line L652 (54.0047, -13.5792) -> (53.2057, -13.5792)
  line L653 (53.2057, -13.5792) -> (53.2057, -7.7792)
  line L654 (53.2057, -7.7792) -> (54.0047, -7.7792)
  line L655 (54.0047, -7.7792) -> (54.0047, -4.6786)
  line L656 (54.0047, -4.6786) -> (53.2057, -4.6786)
  line L657 (53.2057, -4.6786) -> (53.2057, -3.6795)
  line L658 (53.2057, -3.6795) -> (39.2057, -3.6795)
  line L659 (20.1557, -3.6795) -> (20.1557, -4.6786)
  line L660 (20.1557, -4.6786) -> (19.3547, -4.6786)
  line L661 (19.3547, -4.6786) -> (19.3547, -7.7792)
  line L662 (19.3547, -7.7792) -> (20.1557, -7.7792)
  line L663 (20.1557, -7.7792) -> (20.1557, -13.5792)
  line L664 (20.1557, -13.5792) -> (19.3547, -13.5792)
  line L665 (19.3547, -13.5792) -> (19.3547, -16.6784)
  line L666 (19.3547, -16.6784) -> (20.1557, -16.6784)
  line L667 (20.1557, -16.6784) -> (20.1557, -17.6788)
  line L668 (20.1557, -17.6788) -> (34.1557, -17.6788)
  line L669 (34.1557, -17.6788) -> (34.1557, -16.6784)
  line L670 (34.1557, -16.6784) -> (34.9547, -16.6784)
  line L671 (34.9547, -16.6784) -> (34.9547, -13.5792)
  line L672 (34.9547, -13.5792) -> (34.1557, -13.5792)
  line L673 (34.1557, -13.5792) -> (34.1557, -7.7792)
  line L674 (34.1557, -7.7792) -> (34.9547, -7.7792)
  line L675 (34.9547, -7.7792) -> (34.9547, -4.6786)
  line L676 (34.9547, -4.6786) -> (34.1557, -4.6786)
  line L677 (34.1557, -4.6786) -> (34.1557, -3.6795)
  line L678 (34.1557, -3.6795) -> (20.1557, -3.6795)
  line L679 (1.1057, -3.6795) -> (1.1057, -4.6786)
  line L680 (1.1057, -4.6786) -> (0.3047, -4.6786)
  line L681 (0.3047, -4.6786) -> (0.3047, -7.7792)
  line L682 (0.3047, -7.7792) -> (1.1057, -7.7792)
  line L683 (1.1057, -7.7792) -> (1.1057, -13.5792)
  line L684 (1.1057, -13.5792) -> (0.3047, -13.5792)
  line L685 (0.3047, -13.5792) -> (0.3047, -16.6784)
  line L686 (0.3047, -16.6784) -> (1.1057, -16.6784)
  line L687 (1.1057, -16.6784) -> (1.1057, -17.6788)
  line L688 (1.1057, -17.6788) -> (15.1057, -17.6788)
  line L689 (15.1057, -17.6788) -> (15.1057, -16.6784)
  line L690 (15.1057, -16.6784) -> (15.9047, -16.6784)
  line L691 (15.9047, -16.6784) -> (15.9047, -13.5792)
  line L692 (15.9047, -13.5792) -> (15.1057, -13.5792)
  line L693 (15.1057, -13.5792) -> (15.1057, -7.7792)
  line L694 (15.1057, -7.7792) -> (15.9047, -7.7792)
  line L695 (15.9047, -7.7792) -> (15.9047, -4.6786)
  line L696 (15.9047, -4.6786) -> (15.1057, -4.6786)
  line L697 (15.1057, -4.6786) -> (15.1057, -3.6795)
  line L698 (15.1057, -3.6795) -> (1.1057, -3.6795)
  line L699 (-17.9443, -3.6795) -> (-17.9443, -4.6786)
  line L700 (-17.9443, -4.6786) -> (-18.7453, -4.6786)
  line L701 (-18.7453, -4.6786) -> (-18.7453, -7.7792)
  line L702 (-18.7453, -7.7792) -> (-17.9443, -7.7792)
  line L703 (-17.9443, -7.7792) -> (-17.9443, -13.5792)
  line L704 (-17.9443, -13.5792) -> (-18.7453, -13.5792)
  line L705 (-18.7453, -13.5792) -> (-18.7453, -16.6784)
  line L706 (-18.7453, -16.6784) -> (-17.9443, -16.6784)
  line L707 (-17.9443, -16.6784) -> (-17.9443, -17.6788)
  line L708 (-17.9443, -17.6788) -> (-3.9443, -17.6788)
  line L709 (-3.9443, -17.6788) -> (-3.9443, -16.6784)
  line L710 (-3.9443, -16.6784) -> (-3.1453, -16.6784)
  line L711 (-3.1453, -16.6784) -> (-3.1453, -13.5792)
  line L712 (-3.1453, -13.5792) -> (-3.9443, -13.5792)
  line L713 (-3.9443, -13.5792) -> (-3.9443, -7.7792)
  line L714 (-3.9443, -7.7792) -> (-3.1453, -7.7792)
  line L715 (-3.1453, -7.7792) -> (-3.1453, -4.6786)
  line L716 (-3.1453, -4.6786) -> (-3.9443, -4.6786)
  line L717 (-3.9443, -4.6786) -> (-3.9443, -3.6795)
  line L718 (-3.9443, -3.6795) -> (-17.9443, -3.6795)
  line L719 (-36.9943, -3.6795) -> (-36.9943, -4.6786)
  line L720 (-36.9943, -4.6786) -> (-37.7953, -4.6786)
  line L721 (-37.7953, -4.6786) -> (-37.7953, -7.7792)
  line L722 (-37.7953, -7.7792) -> (-36.9943, -7.7792)
  line L723 (-36.9943, -7.7792) -> (-36.9943, -13.5792)
  line L724 (-36.9943, -13.5792) -> (-37.7953, -13.5792)
  line L725 (-37.7953, -13.5792) -> (-37.7953, -16.6784)
  line L726 (-37.7953, -16.6784) -> (-36.9943, -16.6784)
  line L727 (-36.9943, -16.6784) -> (-36.9943, -17.6788)
  line L728 (-36.9943, -17.6788) -> (-22.9943, -17.6788)
  line L729 (-22.9943, -17.6788) -> (-22.9943, -16.6784)
  line L730 (-22.9943, -16.6784) -> (-22.1953, -16.6784)
  line L731 (-22.1953, -16.6784) -> (-22.1953, -13.5792)
  line L732 (-22.1953, -13.5792) -> (-22.9943, -13.5792)
  line L733 (-22.9943, -13.5792) -> (-22.9943, -7.7792)
  line L734 (-22.9943, -7.7792) -> (-22.1953, -7.7792)
  line L735 (-22.1953, -7.7792) -> (-22.1953, -4.6786)
  line L736 (-22.1953, -4.6786) -> (-22.9943, -4.6786)
  line L737 (-22.9943, -4.6786) -> (-22.9943, -3.6795)
  line L738 (-22.9943, -3.6795) -> (-36.9943, -3.6795)
  line L739 (-56.0441, -3.6795) -> (-56.0441, -4.6786)
  line L740 (-56.0441, -4.6786) -> (-56.8449, -4.6786)
  line L741 (-56.8449, -4.6786) -> (-56.8449, -7.7792)
  line L742 (-56.8449, -7.7792) -> (-56.0441, -7.7792)
  line L743 (-56.0441, -7.7792) -> (-56.0441, -13.5792)
  line L744 (-56.0441, -13.5792) -> (-56.8449, -13.5792)
  line L745 (-56.8449, -13.5792) -> (-56.8449, -16.6784)
  line L746 (-56.8449, -16.6784) -> (-56.0441, -16.6784)
  line L747 (-56.0441, -16.6784) -> (-56.0441, -17.6788)
  line L748 (-56.0441, -17.6788) -> (-42.0443, -17.6788)
  line L749 (-42.0443, -17.6788) -> (-42.0443, -16.6784)
  line L750 (-42.0443, -16.6784) -> (-41.2453, -16.6784)
  line L751 (-41.2453, -16.6784) -> (-41.2453, -13.5792)
  line L752 (-41.2453, -13.5792) -> (-42.0443, -13.5792)
  line L753 (-42.0443, -13.5792) -> (-42.0443, -7.7792)
  line L754 (-42.0443, -7.7792) -> (-41.2453, -7.7792)
  line L755 (-41.2453, -7.7792) -> (-41.2453, -4.6786)
  line L756 (-41.2453, -4.6786) -> (-42.0443, -4.6786)
  line L757 (-42.0443, -4.6786) -> (-42.0443, -3.6795)
  line L758 (-42.0443, -3.6795) -> (-56.0441, -3.6795)
  line L759 (-75.0941, -3.6795) -> (-75.0941, -4.6786)
  line L760 (-75.0941, -4.6786) -> (-75.8949, -4.6786)
  line L761 (-75.8949, -4.6786) -> (-75.8949, -7.7792)
  line L762 (-75.8949, -7.7792) -> (-75.0941, -7.7792)
  line L763 (-75.0941, -7.7792) -> (-75.0941, -13.5792)
  line L764 (-75.0941, -13.5792) -> (-75.8949, -13.5792)
  line L765 (-75.8949, -13.5792) -> (-75.8949, -16.6784)
  line L766 (-75.8949, -16.6784) -> (-75.0941, -16.6784)
  line L767 (-75.0941, -16.6784) -> (-75.0941, -17.6788)
  line L768 (-75.0941, -17.6788) -> (-61.0948, -17.6788)
  line L769 (-61.0948, -17.6788) -> (-61.0948, -16.6784)
  line L770 (-61.0948, -16.6784) -> (-60.2954, -16.6784)
  line L771 (-60.2954, -16.6784) -> (-60.2954, -13.5792)
  line L772 (-60.2954, -13.5792) -> (-61.0948, -13.5792)
  line L773 (-61.0948, -13.5792) -> (-61.0948, -7.7792)
  line L774 (-61.0948, -7.7792) -> (-60.2954, -7.7792)
  line L775 (-60.2954, -7.7792) -> (-60.2954, -4.6786)
  line L776 (-60.2954, -4.6786) -> (-61.0948, -4.6786)
  line L777 (-61.0948, -4.6786) -> (-61.0948, -3.6795)
  line L778 (-61.0948, -3.6795) -> (-75.0941, -3.6795)
  line L779 (-94.1441, -3.6795) -> (-94.1441, -4.6786)
  line L780 (-94.1441, -4.6786) -> (-94.9449, -4.6786)
  line L781 (-94.9449, -4.6786) -> (-94.9449, -7.7792)
  line L782 (-94.9449, -7.7792) -> (-94.1441, -7.7792)
  line L783 (-94.1441, -7.7792) -> (-94.1441, -13.5792)
  line L784 (-94.1441, -13.5792) -> (-94.9449, -13.5792)
  line L785 (-94.9449, -13.5792) -> (-94.9449, -16.6784)
  line L786 (-94.9449, -16.6784) -> (-94.1441, -16.6784)
  line L787 (-94.1441, -16.6784) -> (-94.1441, -17.6788)
  line L788 (-94.1441, -17.6788) -> (-80.1448, -17.6788)
  line L789 (-80.1448, -17.6788) -> (-80.1448, -16.6784)
  line L790 (-80.1448, -16.6784) -> (-79.3454, -16.6784)
  line L791 (-79.3454, -16.6784) -> (-79.3454, -13.5792)
  line L792 (-79.3454, -13.5792) -> (-80.1448, -13.5792)
  line L793 (-80.1448, -13.5792) -> (-80.1448, -7.7792)
  line L794 (-80.1448, -7.7792) -> (-79.3454, -7.7792)
  line L795 (-79.3454, -7.7792) -> (-79.3454, -4.6786)
  line L796 (-79.3454, -4.6786) -> (-80.1448, -4.6786)
  line L797 (-80.1448, -4.6786) -> (-80.1448, -3.6795)
  line L798 (-80.1448, -3.6795) -> (-94.1441, -3.6795)
  line L799 (-113.1941, -3.6795) -> (-113.1941, -4.6786)
  line L800 (-113.1941, -4.6786) -> (-113.9948, -4.6786)
  line L801 (-113.9948, -4.6786) -> (-113.9948, -7.7792)
  line L802 (-113.9948, -7.7792) -> (-113.1941, -7.7792)
  line L803 (-113.1941, -7.7792) -> (-113.1941, -13.5792)
  line L804 (-113.1941, -13.5792) -> (-113.9948, -13.5792)
  line L805 (-113.9948, -13.5792) -> (-113.9948, -16.6784)
  line L806 (-113.9948, -16.6784) -> (-113.1941, -16.6784)
  line L807 (-113.1941, -16.6784) -> (-113.1941, -17.6788)
  line L808 (-113.1941, -17.6788) -> (-99.1948, -17.6788)
  line L809 (-99.1948, -17.6788) -> (-99.1948, -16.6784)
  line L810 (-99.1948, -16.6784) -> (-98.3954, -16.6784)
  line L811 (-98.3954, -16.6784) -> (-98.3954, -13.5792)
  line L812 (-98.3954, -13.5792) -> (-99.1948, -13.5792)
  line L813 (-99.1948, -13.5792) -> (-99.1948, -7.7792)
  line L814 (-99.1948, -7.7792) -> (-98.3954, -7.7792)
  line L815 (-98.3954, -7.7792) -> (-98.3954, -4.6786)
  line L816 (-98.3954, -4.6786) -> (-99.1948, -4.6786)
  line L817 (-99.1948, -4.6786) -> (-99.1948, -3.6795)
  line L818 (-99.1948, -3.6795) -> (-113.1941, -3.6795)
  line L819 (-139.3893, -3.6795) -> (-139.3893, -4.6786)
  line L820 (-139.3893, -4.6786) -> (-140.1885, -4.6786)
  line L821 (-140.1885, -4.6786) -> (-140.1885, -7.7792)
  line L822 (-140.1885, -7.7792) -> (-139.3893, -7.7792)
  line L823 (-139.3893, -7.7792) -> (-139.3893, -13.5792)
  line L824 (-139.3893, -13.5792) -> (-140.1885, -13.5792)
  line L825 (-140.1885, -13.5792) -> (-140.1885, -16.6784)
  line L826 (-140.1885, -16.6784) -> (-139.3893, -16.6784)
  line L827 (-139.3893, -16.6784) -> (-139.3893, -17.6788)
  line L828 (-139.3893, -17.6788) -> (-125.3884, -17.6788)
  line L829 (-125.3884, -17.6788) -> (-125.3884, -16.6784)
  line L830 (-125.3884, -16.6784) -> (-124.5891, -16.6784)
  line L831 (-124.5891, -16.6784) -> (-124.5891, -13.5792)
  line L832 (-124.5891, -13.5792) -> (-125.3884, -13.5792)
  line L833 (-125.3884, -13.5792) -> (-125.3884, -7.7792)
  line L834 (-125.3884, -7.7792) -> (-124.5891, -7.7792)
  line L835 (-124.5891, -7.7792) -> (-124.5891, -4.6786)
  line L836 (-124.5891, -4.6786) -> (-125.3884, -4.6786)
  line L837 (-125.3884, -4.6786) -> (-125.3884, -3.6795)
  line L838 (-125.3884, -3.6795) -> (-139.3893, -3.6795)
  line L839 (143.9807, 15.3705) -> (143.9807, 14.3714)
  line L840 (143.9807, 14.3714) -> (143.1797, 14.3714)
  line L841 (143.1797, 14.3714) -> (143.1797, 11.2708)
  line L842 (143.1797, 11.2708) -> (143.9807, 11.2708)
  line L843 (143.9807, 11.2708) -> (143.9807, 5.4708)
  line L844 (143.9807, 5.4708) -> (143.1797, 5.4708)
  line L845 (143.1797, 5.4708) -> (143.1797, 2.3716)
  line L846 (143.1797, 2.3716) -> (143.9807, 2.3716)
  line L847 (143.9807, 2.3716) -> (143.9807, 1.3712)
  line L848 (143.9807, 1.3712) -> (157.9807, 1.3712)
  line L849 (157.9807, 1.3712) -> (157.9807, 2.3716)
  line L850 (157.9807, 2.3716) -> (158.7797, 2.3716)
  line L851 (158.7797, 2.3716) -> (158.7797, 5.4708)
  line L852 (158.7797, 5.4708) -> (157.9807, 5.4708)
  line L853 (157.9807, 5.4708) -> (157.9807, 11.2708)
  line L854 (157.9807, 11.2708) -> (158.7797, 11.2708)
  line L855 (158.7797, 11.2708) -> (158.7797, 14.3714)
  line L856 (158.7797, 14.3714) -> (157.9807, 14.3714)
  line L857 (157.9807, 14.3714) -> (157.9807, 15.3705)
  line L858 (157.9807, 15.3705) -> (143.9807, 15.3705)
  line L859 (115.4057, 15.3705) -> (115.4057, 14.3714)
  line L860 (115.4057, 14.3714) -> (114.6047, 14.3714)
  line L861 (114.6047, 14.3714) -> (114.6047, 11.2708)
  line L862 (114.6047, 11.2708) -> (115.4057, 11.2708)
  line L863 (115.4057, 11.2708) -> (115.4057, 5.4708)
  line L864 (115.4057, 5.4708) -> (114.6047, 5.4708)
  line L865 (114.6047, 5.4708) -> (114.6047, 2.3716)
  line L866 (114.6047, 2.3716) -> (115.4057, 2.3716)
  line L867 (115.4057, 2.3716) -> (115.4057, 1.3712)
  line L868 (115.4057, 1.3712) -> (129.4057, 1.3712)
  line L869 (129.4057, 1.3712) -> (129.4057, 2.3716)
  line L870 (129.4057, 2.3716) -> (130.2047, 2.3716)
  line L871 (130.2047, 2.3716) -> (130.2047, 5.4708)
  line L872 (130.2047, 5.4708) -> (129.4057, 5.4708)
  line L873 (129.4057, 5.4708) -> (129.4057, 11.2708)
  line L874 (129.4057, 11.2708) -> (130.2047, 11.2708)
  line L875 (130.2047, 11.2708) -> (130.2047, 14.3714)
  line L876 (130.2047, 14.3714) -> (129.4057, 14.3714)
  line L877 (129.4057, 14.3714) -> (129.4057, 15.3705)
  line L878 (129.4057, 15.3705) -> (115.4057, 15.3705)
  line L879 (91.5937, 15.3705) -> (91.5937, 14.3714)
  line L880 (91.5937, 14.3714) -> (90.7927, 14.3714)
  line L881 (90.7927, 14.3714) -> (90.7927, 11.2708)
  line L882 (90.7927, 11.2708) -> (91.5937, 11.2708)
  line L883 (91.5937, 11.2708) -> (91.5937, 5.4708)
  line L884 (91.5937, 5.4708) -> (90.7927, 5.4708)